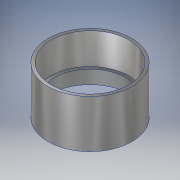
# Autodesk Inventor part: Skirt Master Sketch
Saved by Autodesk Inventor 2017 (Build 210142000, 142)
## iProperties
Created: 2016-07-25
Part Number: Skirt Master Sketch
Material: Aluminum 6061
Document SubType Name: Modeling
Designer: Bill
Density: 2.7 g/cm^3
Appearance: Aluminum - Flat
Author: Bill
Autodesk Inventor part; units mm, degrees
ref_plane "YZ Plane" through (0, 0, 0) normal (1, 0, 0) x (0, 1, 0)
ref_plane "XZ Plane" through (0, 0, 0) normal (0, 1, 0) x (-1, 0, 0)
ref_plane "XY Plane" through (0, 0, 0) normal (0, 0, 1) x (1, 0, 0)
sketch "Sketch1" plane through (0, 0, 0) normal (0, 0, 1) x (1, 0, 0)
  line L0 (-82.55, 51.698) -> (-82.55, -14.3542)
  line L1 (-82.55, -14.3542) -> (-76.2, -14.3542)
  line L2 (-76.2, -14.3542) -> (-85.725, -49.902)
  line L3 (-85.725, -49.902) -> (-88.9, -49.902)
  line L4 (-88.9, -49.902) -> (-88.9, 51.698)
  line L5 (-88.9, 51.698) -> (-82.55, 51.698)
  line L6 (0, -70.222) -> (0, 72.018) projected
  point P0 (0, 0)
  dimension "d0" = 6.35
  dimension "d1" = 3.175
  dimension "d2" = 105
  dimension "d3" = 76.2
  dimension "d4" = 6.35
  dimension "d6" = 101.6
  constraints: 12 end point, 2 perpendicular, 2 vertical, 1 parallel
  measures "d0" distance of L0.end L1.end
  measures "d1" distance of L2.end L3.end
  measures "d2" angle of L3 L2
  measures "d3" horizontal distance of L1.end point (0, 0)
  measures "d4" distance of L4.end L0.start
  measures "d6" distance of L3.end L4.end
revolve "Revolution1" add sketch "Sketch1" angle 360 about axis through (0, -10, 0) along (0, 1, 0)
body "Solid1"
